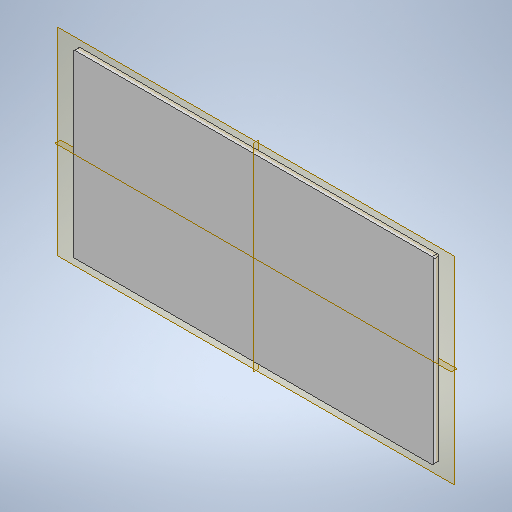
# Autodesk Inventor part: sessao_07_04_002_001
Saved by Autodesk Inventor 2026 (Build 300175000, 175)
## iProperties
Created: 2025-04-07
Part Number: sessao_07_04_002_001
Material: Generic
Document SubType Name: Modeling
Designer: Carlos Dias
Density: 1 g/cm^3
Appearance: Default
Author: Carlos Dias
Autodesk Inventor part; units mm, degrees
sketch "Sketch1" plane through (0, 0, 0) normal (0, 0, 1) x (1, 0, 0)
  line L0 (-250, 125) -> (250, 125)
  line L1 (250, 125) -> (250, -125)
  line L2 (250, -125) -> (-250, -125)
  line L3 (-250, -125) -> (-250, 125)
  line L4 (-250, 125) -> (250, -125) construction
  line L5 (250, 125) -> (-250, -125) construction
  point P0 (0, 0)
  point P1 (0, 0)
  dimension "d0" = 500
  dimension "d1" = 250
  constraints: 12 end point, 2 midpoint, 2 parallel, 1 coincident, 1 horizontal, 1 perpendicular
  measures "d0" distance of L0.start L0.end
  measures "d1" distance of L2.end L0.start
extrude "Extrusion1" add sketch "Sketch1" along normal mid plane 7
fillet "Fillet1" radius 2 4 edges at (250, 125, 0) (-250, 125, 0) (-250, -125, 0) (250, -125, 0)
body "Solid1"
